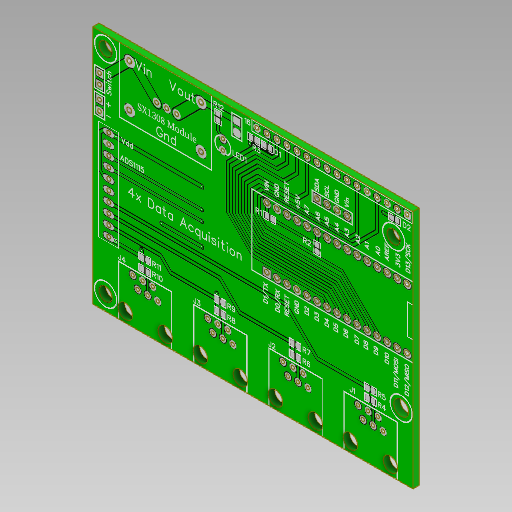
# Autodesk Inventor part: PCB
Saved by Autodesk Inventor 2020 (Build 240168000, 168)
## iProperties
Created: 2019-09-04
Part Number: PCB
Material: Generic
Document SubType Name: Modeling
Designer: amsmi
Density: 1 g/cm^3
Appearance: Default
Author: amsmi
Autodesk Inventor part; units mm, degrees
ref_plane "YZ Plane" through (0, 0, 0) normal (1, 0, 0) x (0, 1, 0)
ref_plane "XZ Plane" through (0, 0, 0) normal (0, 1, 0) x (-1, 0, 0)
ref_plane "XY Plane" through (0, 0, 0) normal (0, 0, 1) x (1, 0, 0)
sketch "Sketch1" plane through (0, 0, 0) normal (0, 0, 1) x (1, 0, 0)
  line L0 (40.64, -30.48) -> (-40.64, -30.48)
  line L1 (-40.64, -30.48) -> (-40.64, 30.48)
  line L2 (-40.64, 30.48) -> (40.64, 30.48)
  line L3 (40.64, 30.48) -> (40.64, -30.48)
  line L4 (40.64, -30.48) -> (-40.64, 30.48) construction
  line L5 (-40.64, -30.48) -> (40.64, 30.48) construction
  point P0 (0, 0)
  dimension "d0" = 81.28
  dimension "d1" = 60.96
  constraints: 12 end point, 2 midpoint, 2 parallel, 1 horizontal, 1 perpendicular
  measures "d0" distance of L1.end L2.end
  measures "d1" distance of L0.end L1.end
extrude "Extrusion1" add sketch "Sketch1" along normal blind 1.5875
sketch "Sketch2" plane through (0, 0, 1.5875) normal (0, 0, 1) x (1, 0, 0)
  line L0 (-40.64, 30.48) -> (40.6513, 30.4649) construction
  line L1 (40.6513, 30.4649) -> (40.64, -30.48) construction
  line L2 (40.64, -30.48) -> (-40.6513, -30.4649) construction
  line L3 (-40.6513, -30.4649) -> (-40.64, 30.48) construction
  point P0 (0, 0)
  point P1 (40.64, -30.48)
  constraints: 1 coincident, 2 other
decal "Decal1"
sketch "Sketch3" plane through (0, 0, 0) normal (0, 0, -1) x (-1, 0, 0)
  line L0 (-40.64, 30.48) -> (40.6513, 30.4649) construction
  line L1 (40.6513, 30.4649) -> (40.64, -30.48) construction
  line L2 (40.64, -30.48) -> (-40.6513, -30.4649) construction
  line L3 (-40.6513, -30.4649) -> (-40.64, 30.48) construction
  point P0 (0, 0)
  point P1 (40.64, -30.48)
  constraints: 1 coincident, 2 other
decal "Decal2"
sketch "Sketch4" plane through (0, 0, 1.5875) normal (0, 0, 1) x (1, 0, 0)
  circle A0 centre (1.016, 29.083) radius 0.508
  circle A1 centre (3.556, 13.843) radius 0.6158
  circle A2 centre (16.3068, 21.1455) radius 0.635
  circle A3 centre (-31.369, 27.6225) radius 0.635
  circle A4 centre (-38.9255, 21.1455) radius 0.508
  circle A5 centre (-36.576, 9.2075) radius 0.508
  circle A6 centre (-30.5117, -19.05) radius 0.4445
  line L0 (40.64, 30.48) -> (-40.64, 30.48) projected
  line L1 (-40.64, 30.48) -> (-40.64, -30.48) projected
  circle A7 centre (6.096, 13.843) radius 0.6158
  circle A8 centre (8.636, 13.843) radius 0.6158
  circle A9 centre (11.176, 13.843) radius 0.6158
  circle A10 centre (13.716, 13.843) radius 0.6158
  circle A11 centre (16.256, 13.843) radius 0.6158
  circle A12 centre (18.796, 13.843) radius 0.6158
  circle A13 centre (21.336, 13.843) radius 0.6158
  circle A14 centre (23.876, 13.843) radius 0.6158
  circle A15 centre (26.416, 13.843) radius 0.6158
  circle A16 centre (28.956, 13.843) radius 0.6158
  circle A17 centre (31.496, 13.843) radius 0.6158
  circle A18 centre (34.036, 13.843) radius 0.6158
  circle A19 centre (36.576, 13.843) radius 0.6158
  circle A20 centre (39.116, 13.843) radius 0.6158
  circle A21 centre (3.556, -1.397) radius 0.6158
  circle A22 centre (6.096, -1.397) radius 0.6158
  circle A23 centre (8.636, -1.397) radius 0.6158
  circle A24 centre (11.176, -1.397) radius 0.6158
  circle A25 centre (13.716, -1.397) radius 0.6158
  circle A26 centre (16.256, -1.397) radius 0.6158
  circle A27 centre (18.796, -1.397) radius 0.6158
  circle A28 centre (21.336, -1.397) radius 0.6158
  circle A29 centre (23.876, -1.397) radius 0.6158
  circle A30 centre (26.416, -1.397) radius 0.6158
  circle A31 centre (28.956, -1.397) radius 0.6158
  circle A32 centre (31.496, -1.397) radius 0.6158
  circle A33 centre (34.036, -1.397) radius 0.6158
  circle A34 centre (36.576, -1.397) radius 0.6158
  circle A35 centre (39.116, -1.397) radius 0.6158
  circle A36 centre (3.556, 29.083) radius 0.508
  circle A37 centre (6.096, 29.083) radius 0.508
  circle A38 centre (8.636, 29.083) radius 0.508
  circle A39 centre (11.176, 29.083) radius 0.508
  circle A40 centre (13.716, 29.083) radius 0.508
  circle A41 centre (16.256, 29.083) radius 0.508
  circle A42 centre (18.796, 29.083) radius 0.508
  circle A43 centre (21.336, 29.083) radius 0.508
  circle A44 centre (23.876, 29.083) radius 0.508
  circle A45 centre (26.416, 29.083) radius 0.508
  circle A46 centre (28.956, 29.083) radius 0.508
  circle A47 centre (31.496, 29.083) radius 0.508
  circle A48 centre (34.036, 29.083) radius 0.508
  circle A49 centre (36.576, 29.083) radius 0.508
  circle A50 centre (39.116, 29.083) radius 0.508
  circle A51 centre (-13.1445, 27.6225) radius 0.635
  circle A52 centre (-31.369, 16.764) radius 0.635
  circle A53 centre (-13.1445, 16.764) radius 0.635
  circle A54 centre (-38.9255, 15.3035) radius 0.508
  circle A55 centre (-38.9255, 18.6055) radius 0.508
  circle A56 centre (-38.9255, 12.7635) radius 0.508
  circle A57 centre (-36.576, 6.6675) radius 0.508
  circle A58 centre (-36.576, 4.1275) radius 0.508
  circle A59 centre (-36.576, 1.5875) radius 0.508
  circle A60 centre (-36.576, -0.9525) radius 0.508
  circle A61 centre (-36.576, -3.4925) radius 0.508
  circle A62 centre (-36.576, -6.0325) radius 0.508
  circle A63 centre (-36.576, -8.5725) radius 0.508
  circle A64 centre (-36.576, -11.1125) radius 0.508
  circle A65 centre (-36.576, -13.6525) radius 0.508
  circle A66 centre (-29.2417, -21.59) radius 0.4445
  circle A67 centre (-27.9717, -19.05) radius 0.4445
  circle A68 centre (-26.7018, -21.59) radius 0.4445
  circle A69 centre (-25.4317, -19.05) radius 0.4445
  circle A70 centre (-24.1617, -21.59) radius 0.4445
  circle A71 centre (-11.4617, -19.05) radius 0.4445
  circle A72 centre (-8.9217, -19.05) radius 0.4445
  circle A73 centre (-6.3817, -19.05) radius 0.4445
  circle A74 centre (-10.1917, -21.59) radius 0.4445
  circle A75 centre (-7.6517, -21.59) radius 0.4445
  circle A76 centre (-5.1117, -21.59) radius 0.4445
  circle A77 centre (7.5883, -19.05) radius 0.4445
  circle A78 centre (10.1283, -19.05) radius 0.4445
  circle A79 centre (12.6683, -19.05) radius 0.4445
  circle A80 centre (8.8583, -21.59) radius 0.4445
  circle A81 centre (11.3983, -21.59) radius 0.4445
  circle A82 centre (13.9383, -21.59) radius 0.4445
  circle A83 centre (26.6382, -19.05) radius 0.4445
  circle A84 centre (29.1783, -19.05) radius 0.4445
  circle A85 centre (31.7183, -19.05) radius 0.4445
  circle A86 centre (27.9082, -21.59) radius 0.4445
  circle A87 centre (30.4482, -21.59) radius 0.4445
  circle A88 centre (32.9883, -21.59) radius 0.4445
  circle A89 centre (-37.4015, 27.2415) radius 1.651
  circle A90 centre (18.8468, 21.1455) radius 0.635
  circle A91 centre (21.3868, 21.1455) radius 0.635
  circle A92 centre (23.9268, 21.1455) radius 0.635
  circle A93 centre (35.687, 22.479) radius 1.651
  circle A94 centre (-32.385, -27.94) radius 1.8415
  line L2 (-40.64, -30.48) -> (40.64, -30.48) projected
  circle A95 centre (-22.225, -27.94) radius 1.8415
  circle A96 centre (-3.175, -27.94) radius 1.8415
  circle A97 centre (-13.335, -27.94) radius 1.8415
  circle A98 centre (15.875, -27.94) radius 1.8415
  circle A99 centre (5.715, -27.94) radius 1.8415
  circle A100 centre (34.925, -27.94) radius 1.8415
  circle A101 centre (24.765, -27.94) radius 1.8415
  circle A102 centre (-37.4015, -26.67) radius 1.651
  circle A103 centre (37.6555, -14.1605) radius 1.905
  line L3 (40.64, -30.48) -> (40.64, 30.48) projected
  circle A104 centre (-7.62, 22.352) radius 0.4445
  circle A105 centre (-7.62, 19.812) radius 0.4445
  circle A106 centre (-24.4221, 21.9075) radius 0.508
  circle A107 centre (-21.8821, 21.9075) radius 0.508
  circle A108 centre (-19.3421, 21.9075) radius 0.508
  point P0 (0, 0)
  dimension "d10" = 1.016
  dimension "d11" = 1.27
  dimension "d12" = 1.016
  dimension "d13" = 1.016
  dimension "d14" = 16.637
  dimension "d15" = 44.196
  dimension "d18" = 2.54
  dimension "d21" = 15.24
  dimension "d24" = 1.397
  dimension "d25" = 41.656
  dimension "d28" = 2.54
  dimension "d33" = 2.8575
  dimension "d34" = 9.271
  dimension "d37" = 18.2245
  dimension "d40" = 10.8585
  dimension "d43" = 1.7145
  dimension "d44" = 9.3345
  dimension "d45" = 5.842
  dimension "d48" = 2.54
  dimension "d53" = 4.064
  dimension "d54" = 21.2725
  dimension "d57" = 2.54
  dimension "d62" = 10.1282
  dimension "d63" = 0.889
  dimension "d64" = 49.53
  dimension "d65" = 1.27
  dimension "d66" = 2.54
  dimension "d69" = 2.54
  dimension "d76" = 19.05
  dimension "d81" = 3.302
  dimension "d82" = 3.2385
  dimension "d83" = 3.2385
  dimension "d84" = 9.3345
  dimension "d85" = 56.9468
  dimension "d86" = 1.27
  dimension "d89" = 2.54
  dimension "d94" = 3.302
  dimension "d95" = 8.001
  dimension "d96" = 76.327
  dimension "d97" = 3.683
  dimension "d98" = 2.54
  dimension "d99" = 8.255
  dimension "d102" = 10.16
  dimension "d109" = 19.05
  dimension "d114" = 3.302
  dimension "d115" = 3.81
  dimension "d116" = 3.81
  dimension "d117" = 2.9845
  dimension "d118" = 16.3195
  dimension "d119" = 0.889
  dimension "d120" = 8.128
  dimension "d121" = 33.02
  dimension "d124" = 2.54
  dimension "d131" = 1.016
  dimension "d132" = 8.5725
  dimension "d133" = 16.2179
  dimension "d136" = 2.54
  constraints: 109 centre point, 9 horizontal, 5 vertical, 2 equal radius, 2 vertical alignment, 187 other
  measures "d10" diameter of A0
  measures "d11" diameter of A3
  measures "d12" diameter of A4
  measures "d13" diameter of A5
  measures "d14" distance from line of L0 A1.centre
  measures "d15" distance from line of L1 A1.centre
  measures "d18" distance of A1.centre A7.centre
  measures "d21" distance of A1.centre A21.centre
  measures "d24" distance from line of L0 A0.centre
  measures "d25" distance from line of L1 A0.centre
  measures "d28" distance of A0.centre A36.centre
  measures "d33" distance from line of L0 A3.centre
  measures "d34" distance from line of L1 A3.centre
  measures "d37" distance of A3.centre A51.centre
  measures "d40" distance of A3.centre A52.centre
  measures "d43" distance from line of L1 A4.centre
  measures "d44" distance from line of L0 A4.centre
  measures "d45" distance of A4.centre A54.centre
  measures "d48" distance of A4.centre A55.centre
  measures "d53" distance from line of L1 A5.centre
  measures "d54" distance from line of L0 A5.centre
  measures "d57" distance of A5.centre A57.centre
  measures "d62" distance from line of L1 A6.centre
  measures "d63" diameter of A6
  measures "d64" distance from line of L0 A6.centre
  measures "d65" horizontal distance of A66.centre A6.centre
  measures "d66" vertical distance of A6.centre A66.centre
  measures "d69" distance of A6.centre A67.centre
  measures "d76" distance of A6.centre A71.centre
  measures "d81" diameter of A89
  measures "d82" distance from line of L1 A89.centre
  measures "d83" distance from line of L0 A89.centre
  measures "d84" distance from line of L0 A2.centre
  measures "d85" distance from line of L1 A2.centre
  measures "d86" diameter of A2
  measures "d89" distance of A2.centre A90.centre
  measures "d94" diameter of A93
  measures "d95" distance from line of L0 A93.centre
  measures "d96" distance from line of L1 A93.centre
  measures "d97" diameter of A94
  measures "d98" distance from line of L2 A94.centre
  measures "d99" distance from line of L1 A94.centre
  measures "d102" distance of A94.centre A95.centre
  measures "d109" distance of A95.centre A96.centre
  measures "d114" diameter of A102
  measures "d115" distance from line of L2 A102.centre
  measures "d116" diameter of A103
  measures "d117" distance from line of L3 A103.centre
  measures "d118" distance from line of L2 A103.centre
  measures "d119" diameter of A104
  measures "d120" distance from line of L0 A104.centre
  measures "d121" distance from line of L1 A104.centre
  measures "d124" distance of A104.centre A105.centre
  measures "d131" diameter of A106
  measures "d132" distance from line of L0 A106.centre
  measures "d133" distance from line of L1 A106.centre
  measures "d136" distance of A106.centre A107.centre
extrude "Extrusion2" cut sketch "Sketch4" against normal through all contours A0 | A1 | A2 | A3 | A4 | A5 | A6 | A7 | A8 | A9 | A10 | A11 | A12 | A13 | A14 | A15 | A16 | A17 | A18 | A19 | A20 | A21 | A22 | A23 | A24 | A25 | A26 | A27 | A28 | A29 | A30 | A31 | A32 | A33 | A34 | A35 | A36 | A37 | A38 | A39 | A40 | A41 | A42 | A43 | A44 | A45 | A46 | A47 | A48 | A49 | A50 | A51 | A52 | A53 | A54 | A55 | A56 | A57 | A58 | A59 | A60 | A61 | A62 | A63 | A64 | A65 | A66 | A67 | A68 | A69 | A70 | A71 | A72 | A73 | A74 | A75 | A76 | A77 | A78 | A79 | A80 | A81 | A82 | A83 | A84 | A85 | A86 | A87 | A88 | A89 | A90 | A91 | A92 | A93 | A94 | A95 | A96 | A97 | A98 | A99 | A100 | A101 | A102 | A103 | A104 | A105 | A106 | A107 | A108
equation "\"d83\" = d82"
body "Solid1"
